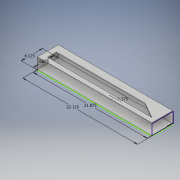
# Autodesk Inventor part: Wire Housing No Support Struct vglue
Saved by Autodesk Inventor 2019 (Build 230136000, 136)
## iProperties
Created: 2020-03-05
Part Number: Wire Housing No Support Struct vglue
Material: Generic
Document SubType Name: Modeling
Designer: Obscure_Decision
Density: 1 g/cm^3
Appearance: Default
Author: Obscure_Decision
Autodesk Inventor part; units mm, degrees
ref_plane "YZ Plane" through (0, 0, 0) normal (1, 0, 0) x (0, 1, 0)
ref_plane "XZ Plane" through (0, 0, 0) normal (0, 1, 0) x (-1, 0, 0)
ref_plane "XY Plane" through (0, 0, 0) normal (0, 0, 1) x (1, 0, 0)
sketch "Sketch1" plane through (0, 0, 0) normal (0, 1, 0) x (-1, 0, 0)
  line L0 (-280.9875, -52.3875) -> (-280.9875, 52.3875)
  line L1 (-280.9875, 52.3875) -> (280.9875, 52.3875)
  line L2 (280.9875, 52.3875) -> (280.9875, -52.3875)
  line L3 (280.9875, -52.3875) -> (-280.9875, -52.3875)
  line L4 (-280.9875, -52.3875) -> (280.9875, 52.3875) construction
  line L5 (-280.9875, 52.3875) -> (280.9875, -52.3875) construction
  line L6 (0, -52.3875) -> (0, -17.4625) construction
  line L7 (-277.8125, -49.2125) -> (277.8125, -49.2125)
  line L8 (277.8125, -49.2125) -> (277.8125, 49.2125)
  line L9 (277.8125, 49.2125) -> (-277.8125, 49.2125) construction
  line L10 (-277.8125, 49.2125) -> (-277.8125, -49.2125)
  line L11 (-277.8125, -49.2125) -> (277.8125, 49.2125) construction
  line L12 (277.8125, -49.2125) -> (-277.8125, 49.2125) construction
  line L13 (277.8125, 49.2125) -> (277.8125, 52.3875)
  line L14 (-277.8125, 49.2125) -> (-277.8125, 52.3875)
  point P0 (0, 0)
  dimension "d0" = 104.775
  dimension "d1" = 561.975
  dimension "d2" = 34.925
  dimension "d3" = 555.625
  dimension "d4" = 98.425
  constraints: 30 end point, 4 parallel, 3 midpoint, 3 perpendicular, 3 point on line, 1 horizontal, 1 vertical
  measures "d0" distance of L1.end L2.end
  measures "d1" distance of L0.end L1.end
  measures "d2" distance of L6.start L6.end
  measures "d3" distance of L9.end L8.end
  measures "d4" distance of L8.end L7.end
extrude "Extrusion1" add sketch "Sketch1" along normal blind 3.175 contours L1 L13 L8 L7 L10 L14
extrude "Extrusion2" add sketch "Sketch1" along normal blind 50.8 contours L0 L1 L14 L10 L7 L8 L13 L2 L3
sketch "Sketch2" plane through (0, 50.8, 0) normal (0, 1, 0) x (1, 0, 0)
  line L0 (-280.9875, -52.3875) -> (-277.8125, -52.3875) projected
  line L1 (-280.9875, -52.3875) -> (255.5875, -52.3875)
  line L2 (280.9875, -52.3875) -> (280.9875, -26.9875)
  line L3 (-280.9875, -26.9875) -> (-280.9875, -52.3875)
  line L4 (-280.9875, 52.3875) -> (-280.9875, -52.3875) projected
  line L5 (-280.9875, 52.3875) -> (255.5875, 52.3875)
  line L6 (280.9875, 52.3875) -> (280.9875, 17.4625)
  line L7 (-280.9875, 17.4625) -> (-280.9875, 52.3875)
  line L8 (-280.9875, 52.3875) -> (-255.5875, 52.3875)
  line L9 (-255.5875, -52.3875) -> (-280.9875, -52.3875)
  line L10 (-280.9875, -52.3875) -> (-280.9875, -26.9875)
  line L11 (-277.8125, -52.3875) -> (277.8125, -52.3875) projected
  line L12 (280.9875, 52.3875) -> (255.5875, 52.3875)
  line L13 (255.5875, -52.3875) -> (280.9875, -52.3875)
  line L14 (280.9875, -52.3875) -> (280.9875, 17.4625)
  line L15 (255.5875, 17.4625) -> (255.5875, -26.9875)
  line L16 (255.5875, 17.4625) -> (-255.5875, 17.4625)
  line L17 (255.5875, 52.3875) -> (280.9875, 52.3875)
  line L18 (280.9875, 17.4625) -> (280.9875, 52.3875)
  line L19 (255.5875, -26.9875) -> (-255.5875, -26.9875)
  line L20 (255.5875, -52.3875) -> (280.9875, -52.3875)
  line L21 (-255.5875, 17.4625) -> (-255.5875, -26.9875)
  line L22 (-280.9875, 17.4625) -> (-280.9875, 52.3875)
  line L23 (-280.9875, -26.9875) -> (-280.9875, 17.4625)
  line L24 (-277.8125, -52.3875) -> (-277.8125, 49.2125) construction
  line L25 (-277.8125, -52.3875) -> (-277.8125, -49.2125) construction
  line L26 (-277.8125, -49.2125) -> (277.8125, -49.2125)
  line L27 (-277.8125, -49.2125) -> (-277.8125, -52.3875)
  line L28 (277.8125, -49.2125) -> (277.8125, -52.3875)
  point P0 (0, 0)
  dimension "d9" = 561.975
  dimension "d10" = 25.4
  dimension "d11" = 561.975
  dimension "d12" = 34.925
  dimension "d13" = 25.4
  dimension "d14" = 104.775
  dimension "d15" = 25.4
  dimension "d18" = 3.175
  dimension "d19" = 555.625
  constraints: 50 end point, 14 parallel, 6 horizontal, 6 perpendicular, 2 point on line, 1 vertical
  measures "d9" distance of L3.start L2.end
  measures "d10" distance of L2.end L2.start
  measures "d11" distance of L6.end L7.start
  measures "d12" distance of L6.start L6.end
  measures "d13" distance of L9.start L9.end
  measures "d14" distance of L8.end L9.start
  measures "d15" distance of L13.end L1.end
  measures "d18" distance of L0.end L25.end
  measures "d19" distance of L25.end L26.end
extrude "Extrusion3" add sketch "Sketch2" along normal blind 3.175
sketch "Sketch3" plane through (0, 53.975, 0) normal (0, 1, 0) x (1, 0, 0)
  line L0 (-277.8125, -52.3875) -> (-277.8125, 49.2125) projected
  line L1 (-277.8125, -52.3875) -> (277.8125, -52.3875)
  line L2 (277.8125, -52.3875) -> (277.8125, -49.2125)
  line L3 (277.8125, -49.2125) -> (-277.8125, -49.2125)
  line L4 (-277.8125, -49.2125) -> (-277.8125, -52.3875)
  point P0 (0, 0)
  dimension "d20" = 555.625
  dimension "d21" = 3.175
  constraints: 8 end point, 2 parallel, 1 horizontal, 1 perpendicular
  measures "d20" distance of L3.end L2.end
  measures "d21" distance of L2.end L1.end
extrude "Extrusion4" cut sketch "Sketch3" against normal blind 3.175
sketch "Sketch4" plane through (280.9875, 0, 52.3875) normal (1, 0, 0) x (0, 0, -1)
  line L0 (3.175, 53.975) -> (0, 53.975) projected
  line L1 (0, 53.975) -> (104.775, 53.975)
  line L2 (104.775, 53.975) -> (104.775, 0)
  line L3 (0, 0) -> (0, 53.975)
  line L4 (52.3875, 0) -> (52.3875, 3.175) construction
  line L5 (0, 3.175) -> (101.6, 3.175) construction
  line L6 (0, 3.175) -> (104.775, 3.175)
  line L7 (104.775, 0) -> (104.775, 53.975) projected
  constraints: 10 end point, 2 perpendicular, 2 point on line, 1 horizontal, 1 parallel, 1 vertical
extrude "Extrusion5" cut sketch "Sketch4" against normal blind 3.175
sketch "Sketch5" plane through (0, 53.975, 0) normal (0, 1, 0) x (1, 0, 0)
  line L0 (255.5875, -26.9875) -> (255.5875, 17.4625) projected
  line L1 (255.5875, -26.9875) -> (178.5978, 17.4625)
  line L2 (255.5875, 17.4625) -> (-255.5875, 17.4625) projected
  line L3 (255.5875, -26.9875) -> (344.4875, -26.9875) construction
  line L4 (178.5978, 17.4625) -> (255.5875, 17.4625)
  point P0 (0, 0)
  dimension "d26" = 150
  constraints: 6 end point, 1 collinear, 1 equal length, 1 horizontal, 1 point on line
  measures "d26" angle of L3 L1
extrude "Extrusion6" add sketch "Sketch5" against normal blind 3.175
sketch "Sketch6" plane through (277.8125, 0, 52.3875) normal (1, 0, 0) x (0, 0, -1)
  line L0 (104.775, 0) -> (104.775, 53.975) projected
  line L1 (104.775, 50.8) -> (104.775, 53.975)
  line L2 (104.775, 53.975) -> (101.6, 53.975)
  line L3 (101.6, 3.175) -> (104.775, 3.175)
  line L4 (104.775, 3.175) -> (104.775, 50.8)
  line L5 (101.6, 50.8) -> (101.6, 3.175)
  line L6 (101.6, 50.8) -> (101.6, 53.975)
  point P0 (52.3875, 0)
  point P1 (3.175, 50.8)
  constraints: 12 end point, 1 horizontal, 1 parallel, 1 perpendicular, 1 point on line, 1 vertical
extrude "Extrusion7" add sketch "Sketch6" along normal blind 3.175
sketch "Sketch8" plane through (0, 3.175, 0) normal (0, 1, 0) x (1, 0, 0)
  line L0 (277.8125, -49.2125) -> (277.8125, 49.2125) projected
  line L1 (277.8125, 49.2125) -> (279.4635, 49.2125)
  line L2 (279.4635, 49.2125) -> (279.4635, 23.6855)
  line L3 (279.4635, 23.6855) -> (277.8125, 23.6855)
  line L4 (277.8125, 23.6855) -> (277.8125, 49.2125)
  point P0 (0, 0)
  dimension "d36" = 1.651
  dimension "d37" = 25.527
  constraints: 8 end point, 2 parallel, 1 horizontal, 1 perpendicular
  measures "d36" distance of L2.end L3.end
  measures "d37" distance of L1.end L2.end
extrude "Extrusion9" cut sketch "Sketch8" against normal blind 3.175
body "Solid1"
